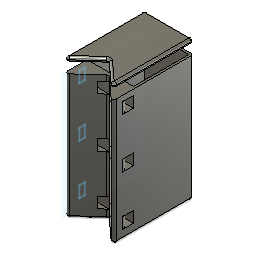
ShakeMap-case v2 (Autodesk Fusion 360 design; units mm, degrees)
Autodesk Fusion 360 part; units mm, degrees
sketch "Sketch1" plane through (0, 0, 0) normal (0, 1, 0) x (1, 0, 0)
  line L0 (0, 0) -> (44, 0)
  line L1 (44, 0) -> (44, -54)
  line L2 (44, -54) -> (0, -54)
  line L3 (0, -54) -> (0, 0)
  line L4 (2, -2) -> (42, -2)
  line L5 (42, -2) -> (42, -52)
  line L6 (42, -52) -> (2, -52)
  line L7 (2, -52) -> (2, -2)
  line L8 (0, -54) -> (0, -74)
  line L9 (0, -74) -> (22, -54)
  line L10 (44, -54) -> (44, -74)
  line L11 (44, -74) -> (22, -54)
  constraint horizontal L0
  constraint vertical L1
  constraint horizontal L2
  constraint vertical L3
  constraint coincident L0.start L3.end
  constraint horizontal L4
  constraint vertical L5
  constraint horizontal L6
  constraint vertical L7
  constraint perpendicular L2 L8
  constraint midpoint L2 L9.end
  constraint perpendicular L2 L10
extrude "Extrude3" add sketch "Sketch1" along normal blind 110 makes body 1
extrude "Extrude4" add sketch "Sketch1" against normal blind 3 contours L0 L1 L2 L3 | L2 L8 L9 | L2 L10 L11 | L4 L5 L6 L7 bodies 1
sketch "Sketch3" plane through (0, 0, 0) normal (-1, 0, 0) x (0, 0, 1)
  line L0 (74, -3) -> (74, 110)
  line L1 (74, 110) -> (0, 110)
  line L2 (0, 110) -> (0, -3)
  line L3 (0, -3) -> (74, -3)
  line L4 (54, 5) -> (59, 5)
  line L5 (59, 5) -> (59, 15)
  line L6 (59, 15) -> (54, 15)
  line L7 (54, 15) -> (54, 5)
  line L8 (54, 50) -> (59, 50)
  line L9 (59, 50) -> (59, 60)
  line L10 (54, 60) -> (54, 50)
  line L11 (59, 60) -> (54, 60)
  line L12 (54, 95) -> (59, 95)
  line L13 (59, 95) -> (59, 105)
  line L14 (54, 105) -> (54, 95)
  line L15 (59, 105) -> (54, 105)
  dimension "d15" = 0
  dimension "d16" = 90
  constraint horizontal L4
  constraint vertical L5
  constraint horizontal L6
  constraint vertical L7
extrude "Extrude5" cut sketch "Sketch3" against normal blind 55 contours L4 L5 L6 L7 | L8 L9 L10 L11 | L12 L13 L14 L15 bodies 1
extrude "Extrude6" add sketch "Sketch1" along normal blind 3 separate body contours L0 L1 L2 L3 | L2 L8 L9 | L2 L10 L11 | L4 L5 L6 L7 makes body 2
extrude "Extrude7" add sketch "Sketch1" against normal blind 2 contours L4 L5 L6 L7 bodies 2
move_body "Move1" bodies 2 to x (1, 0, 0) y (0, 1, 0) z (0, 0, 1) at (0, 110, 0)
fillet "Fillet1" radius 5 6 edges at (0, 100, 59) (0, 55, 59) (0, 10, 59) (44, 100, 59) (44, 55, 59) (44, 10, 59) on bodies 1
fillet "Fillet2" radius 2 10 edges at (22, 113, 0) (44, 113, 37) (33, 113, 64) (11, 113, 64) (0, 113, 37) (0, 111.5, 74) (22, 111.5, 54) (44, 111.5, 74) (44, 111.5, 0) (0, 111.5, 0) on bodies 2
fillet "Fillet3" radius 2 8 edges at (0, 53.5, 74) (22, 77.5, 54) (44, 53.5, 74) (44, 53.5, 0) (22, 107.5, 54) (22, 32.5, 54) (22, 1, 54) (0, 53.5, 0) on bodies 1
fillet "Fillet3" radius 2 5 edges at (0, -3, 37) (11, -3, 64) (33, -3, 64) (44, -3, 37) (22, -3, 0) on bodies 1
move_body "Move2" bodies 2 to x (1, 0, 0) y (0, 1, 0) z (0, 0, 1) at (0, 10, 0)
named bodies: "case", "case-lid"
